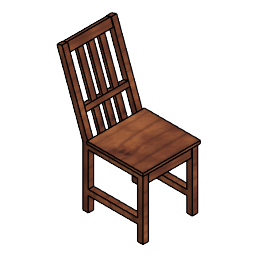
Wooden_chair (Autodesk Fusion 360 design; units mm, degrees)
part number: 2026-07-13-20-45-55-122
Autodesk Fusion 360 part; units mm, degrees
note: some values were not read from the file. Set by a fixed rule: which face or edge a step refers to.
sketch "Sketch1" plane through (0, 0, 0) normal (0, 1, 0) x (1, 0, 0)
  line L0 (0, 0) -> (0, -44)
  line L1 (0, -44) -> (-19.1531, -96.6228)
  line L2 (0, -44) -> (56, -44) construction
  line L3 (-4, 0) -> (-4, -43.2947)
  line L4 (-4, -43.2947) -> (-22.9119, -95.2547)
  line L5 (0, 0) -> (-4, 0)
  line L6 (-19.1531, -96.6228) -> (-22.9119, -95.2547)
  line L7 (40, 0) -> (40, -44)
  line L8 (36, 0) -> (36, -44)
  line L9 (40, 0) -> (36, 0)
  line L10 (0, -40) -> (36, -40)
  line L11 (0, -15) -> (36, -15)
  line L12 (36, -15) -> (36, -11)
  line L13 (36, -11) -> (0, -11)
  line L14 (0, -11) -> (0, -15)
  line L15 (40, -44) -> (0, -44)
  line L16 (0, -40) -> (0, -15)
  line L17 (0, -44) -> (0, -40)
  line L18 (0, -15) -> (0, -11)
  line L19 (36, -15) -> (36, -11)
  line L20 (36, -15) -> (36, -11)
  dimension "d1" = 44
  dimension "d2" = 110
  dimension "d3" = 56
  dimension "d4" = 4
  dimension "d5" = 44
  dimension "d6" = 4
  dimension "d7" = 4
  dimension "d8" = 11
  constraint coincident L0.start L5.start
  constraint vertical L0
  constraint horizontal L2
  constraint perpendicular L3 L5
  constraint perpendicular L4 L6
  constraint vertical L7
  constraint perpendicular L8 L9
  constraint perpendicular L0 L2
  constraint coincident L2 L8.end
  constraint coincident L0 L10.start
  constraint coincident L8 L10.end
  constraint perpendicular L8 L10
  constraint horizontal L11
  constraint vertical L12
  constraint horizontal L13
  constraint vertical L14
  constraint coincident L0 L11.start
  constraint perpendicular L0 L15
  measures "d1" distance of L0.start L0.end
  measures "d2" angle of L1 L2
  measures "d3" distance of L0.end L1.end
  measures "d5" distance of L7.end L7.start
  measures "d6" distance of L2 L10
  measures "d7" distance of L11.start L13.end
  measures "d8" distance of L0.start L13
extrude "Extrude1" add sketch "Sketch1" along normal blind 4 contours L0 L1 L3 L4 L5 L6 L14 L16 L17 L18 | L0 L8 L11 L12 L13 L14 L18 L19 L20 | L7 L8 L9 L12 L15 L19 L20 | L0 L8 L10 L15 L17 makes body 1
copy_body "CopyPasteBodies1" bodies 1 makes body 2
move_body "Move1" bodies 2 to x (1, 0, 0) y (0, 1, 0) z (0, 0, 1) at (0, 36, 0)
sketch "Sketch2" plane through (0, 36, 0) normal (0, -1, 0) x (1, 0, 0)
  line L0 (0, 40) -> (36, 40)
  line L1 (36, 40) -> (36, 15)
  line L2 (36, 15) -> (0, 15)
  line L3 (0, 15) -> (0, 40)
  line L4 (36, 0) -> (40, 0)
  line L5 (40, 0) -> (40, 44)
  line L6 (40, 44) -> (0, 44)
  line L7 (0, 44) -> (-19.1531, 96.6228)
  line L8 (-19.1531, 96.6228) -> (-22.9119, 95.2547)
  line L9 (-22.9119, 95.2547) -> (-4, 43.2947)
  line L10 (-4, 43.2947) -> (-4, 0)
  line L11 (-4, 0) -> (0, 0)
  line L12 (0, 0) -> (0, 11)
  line L13 (0, 11) -> (36, 11)
  line L14 (36, 11) -> (36, 0)
  line L15 (36.5, 42.7055) -> (39.5, 42.7055)
  line L16 (39.5, 42.7055) -> (39.5, 36.7055)
  line L17 (39.5, 36.7055) -> (36.5, 36.7055)
  line L18 (36.5, 36.7055) -> (36.5, 42.7055)
  dimension "d11" = 3
  dimension "d12" = 6
  dimension "d13" = 0.5
  constraint horizontal L15
  constraint vertical L16
  constraint horizontal L17
  constraint vertical L18
  measures "d11" distance of L15.start L15.end
  measures "d12" distance of L15.start L17.end
  measures "d13" distance of L1 L18
extrude "Extrude2" add sketch "Sketch2" along normal blind 32 separate body contours L15 L16 L17 L18 makes body 3
sketch "Sketch3" plane through (0, 0, 44) normal (0, 0, 1) x (-1, 0, 0)
  line L0 (0, 0) -> (-40, 0)
  line L1 (-40, 0) -> (-40, -4)
  line L2 (-40, -4) -> (0, -4)
  line L3 (0, -4) -> (0, 0)
  line L4 (0, 0) -> (-40, -40)
  line L5 (-40, -41) -> (0, -41)
  line L6 (0, -41) -> (0, 1)
  line L7 (0, 1) -> (-40, 1)
  line L8 (-40, 1) -> (-40, -41)
  line L9 (-40, -41) -> (0, 1) construction
  line L10 (0, -41) -> (-40, 1) construction
  point P0 (-40, -40)
  point P1 (-20, -20)
  point P2 (-20, -20)
  dimension "d16" = 40
  dimension "d17" = 42
  constraint coincident L0.start L3.end
  constraint coincident P0 L4.end
  constraint midpoint L4 P2
  constraint horizontal L5
  constraint perpendicular L5 L6
  constraint parallel L5 L7
  constraint parallel L6 L8
  constraint coincident L9 P2
  constraint coincident L10 P2
  constraint coincident P2 P1
  measures "d16" distance of L6.end L7.end
  measures "d17" distance of L5.end L6.end
extrude "Extrude3" add sketch "Sketch3" along normal blind 2 separate body makes body 4
extrude "Extrude4" add 4 faces at (40, 1.3333, 44.6667) (40, 16, 44.6667) (40, 40.3333, 44.6667) (40, -0.6667, 44.6667) along direction (1, 0, 0) blind 1 on bodies 4 bodies 1 3 4 2
sketch "Sketch4" plane through (0, 36, 0) normal (0, -1, 0) x (1, 0, 0)
  line L0 (0, 40) -> (36, 40)
  line L1 (36, 40) -> (36, 15)
  line L2 (36, 15) -> (0, 15)
  line L3 (0, 15) -> (0, 40)
  line L4 (36, 0) -> (40, 0)
  line L5 (40, 0) -> (40, 44)
  line L6 (40, 44) -> (0, 44)
  line L7 (0, 44) -> (-19.1531, 96.6228)
  line L8 (-19.1531, 96.6228) -> (-22.9119, 95.2547)
  line L9 (-22.9119, 95.2547) -> (-4, 43.2947)
  line L10 (-4, 43.2947) -> (-4, 0)
  line L11 (-4, 0) -> (0, 0)
  line L12 (0, 0) -> (0, 11)
  line L13 (0, 11) -> (36, 11)
  line L14 (36, 11) -> (36, 0)
  line L15 (-22.4421, 95.4257) -> (-20.3899, 89.7876)
  line L16 (-19.623, 96.4518) -> (-17.5709, 90.8136)
  line L17 (-20.3899, 89.7876) -> (-17.5709, 90.8136)
  dimension "d22" = 6
  dimension "d23" = -3
  dimension "d24" = 0.5
  constraint coincident L8 L15.start
  constraint perpendicular L8 L15
  constraint perpendicular L16 L17
  measures "d22" distance of L15.start L15.end
  measures "d24" distance of L9 L15
extrude "Extrude5" add sketch "Sketch4" along normal blind 32 separate body contours L8 L15 L16 L17 makes body 5
sketch "Sketch5" plane through (0, 36, 0) normal (0, -1, 0) x (1, 0, 0)
  line L0 (0, 40) -> (36, 40)
  line L1 (36, 40) -> (36, 15)
  line L2 (36, 15) -> (0, 15)
  line L3 (0, 15) -> (0, 40)
  line L4 (36, 0) -> (40, 0)
  line L5 (40, 0) -> (40, 44)
  line L6 (40, 44) -> (0, 44)
  line L7 (0, 44) -> (-19.1531, 96.6228)
  line L8 (-19.1531, 96.6228) -> (-22.9119, 95.2547)
  line L9 (-22.9119, 95.2547) -> (-4, 43.2947)
  line L10 (-4, 43.2947) -> (-4, 0)
  line L11 (-4, 0) -> (0, 0)
  line L12 (0, 0) -> (0, 11)
  line L13 (0, 11) -> (36, 11)
  line L14 (36, 11) -> (36, 0)
  line L15 (-10.4866, 61.1166) -> (-6.7279, 62.4846)
  line L16 (-9.2814, 57.8054) -> (-5.5227, 59.1734)
  constraint coincident L9 L15.start
  constraint coincident L7 L15.end
  constraint perpendicular L7 L15
  constraint coincident L9 L16.start
  constraint coincident L7 L16.end
  constraint perpendicular L7 L16
extrude "Extrude6" add sketch "Sketch5" along normal blind 32 separate body contours L7 L9 L15 L16 makes body 6
sketch "Sketch6" plane through (-20.8692, 0, 57.3376) normal (-0.34202, 0, 0.939693) x (0, -1, 0)
  line L0 (-36, 15.0489) -> (-36, 11.0489)
  line L1 (-36, 11.0489) -> (-4, 11.0489)
  line L2 (-4, 11.0489) -> (-4, 15.0489)
  line L3 (-4, 15.0489) -> (-36, 15.0489)
  line L4 (-18, 14.0489) -> (-22, 14.0489)
  line L5 (-22, 14.0489) -> (-22, 12.0489)
  line L6 (-22, 12.0489) -> (-18, 12.0489)
  line L7 (-18, 12.0489) -> (-18, 14.0489)
  line L8 (-18, 14.0489) -> (-22, 12.0489) construction
  line L9 (-22, 14.0489) -> (-18, 12.0489) construction
  line L10 (-10, 12.0489) -> (-10, 14.0489)
  line L11 (-14, 14.0489) -> (-14, 12.0489)
  line L12 (-14, 12.0489) -> (-10, 12.0489)
  line L13 (-10, 14.0489) -> (-14, 12.0489) construction
  line L14 (-10, 14.0489) -> (-14, 14.0489)
  line L15 (-14, 14.0489) -> (-10, 12.0489) construction
  line L16 (-26, 14.0489) -> (-30, 14.0489)
  line L17 (-26, 14.0489) -> (-30, 12.0489) construction
  line L18 (-30, 14.0489) -> (-30, 12.0489)
  line L19 (-26, 12.0489) -> (-26, 14.0489)
  line L20 (-30, 12.0489) -> (-26, 12.0489)
  line L21 (-30, 14.0489) -> (-26, 12.0489) construction
  point P0 (-4, 11.0489)
  point P1 (-36, 15.0489)
  point P2 (-20, 13.0489)
  point P3 (-20, 13.0489)
  point P4 (-12, 13.0489)
  point P5 (-12, 13.0489)
  point P6 (-28, 13.0489)
  point P7 (-28, 13.0489)
  dimension "d29" = 4
  dimension "d30" = 2
  dimension "d31" = 4
  dimension "d32" = 2
  dimension "d33" = 4
  dimension "d34" = 2
  dimension "d35" = 4
  dimension "d36" = 4
  constraint horizontal L4
  constraint perpendicular L4 L5
  constraint parallel L4 L6
  constraint parallel L5 L7
  constraint coincident L8 P3
  constraint coincident L9 P3
  constraint coincident P3 P2
  constraint horizontal L14
  constraint perpendicular L11 L14
  constraint parallel L12 L14
  constraint parallel L10 L11
  constraint coincident P5 L13
  constraint coincident P5 L15
  constraint coincident P5 P4
  constraint horizontal L16
  constraint perpendicular L16 L18
  constraint parallel L16 L20
  constraint parallel L18 L19
  constraint coincident P7 L17
  constraint coincident P7 L21
  constraint coincident P7 P6
  measures "d29" distance of L5.end L6.end
  measures "d30" distance of L4.end L5.end
  measures "d31" distance of L11.end L10.start
  measures "d32" distance of L11.start L11.end
  measures "d33" distance of L17.end L19.start
  measures "d34" distance of L16.end L17.end
  measures "d35" distance of L5 L19
  measures "d36" distance of L7 L11
extrude "Extrude7" add sketch "Sketch6" along normal blind 30 and the other way blind 20 separate body contours L4 L5 L6 L7 | L10 L11 L12 L14 | L16 L18 L19 L20 makes body 7 at (-8.4069, 12.6667, 58.3263) makes body 8 at (-8.4069, 20.6667, 58.3263) makes body 9 at (-8.4069, 28.6667, 58.3263)
